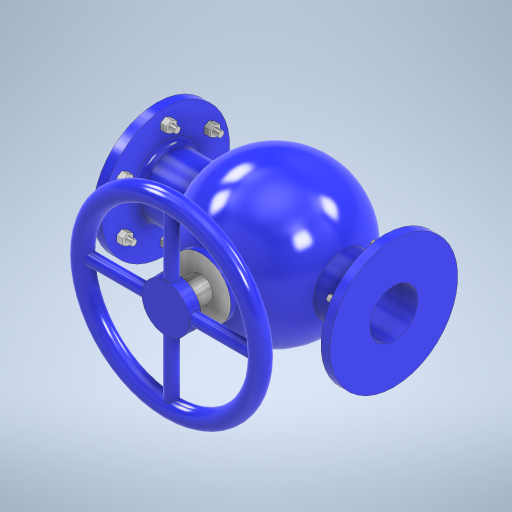
# Autodesk Inventor part: Flansch DN80
Saved by Autodesk Inventor 2023 (Build 270158000, 158)
## iProperties
Created: 2024-11-14
Part Number: Flansch DN80
Material: Generisch
Document SubType Name: Modeling
Designer: aurich
Density: 1 g/cm^3
Appearance: Vorgabe
Author: aurich
Autodesk Inventor part; units mm, degrees
ref_plane "YZ Plane" through (0, 0, 0) normal (1, 0, 0) x (0, 1, 0)
ref_plane "XZ Plane" through (0, 0, 0) normal (0, 1, 0) x (-1, 0, 0)
sketch "Skizze1" plane through (0, 0, 0) normal (1, 0, 0) x (0, 1, 0)
  circle A0 centre (0, 0) radius 40
  circle A1 centre (0, 0) radius 108
  dimension "d0" = 216
  dimension "d1" = 80
  constraints: 2 centre point, 2 coincident
  measures "d0" diameter of A1
  measures "d1" diameter of A0
extrude "Extrusion1" add sketch "Skizze1" along normal blind 15
sketch "Skizze2" plane through (15, 0, 0) normal (1, 0, 0) x (0, 0, -1)
  circle A0 centre (0, 0) radius 40
  circle A1 centre (0, 0) radius 50
  dimension "d4" = 100
  constraints: 2 centre point, 2 coincident
  measures "d4" diameter of A1
extrude "Extrusion2" add sketch "Skizze2" along normal blind 185
fillet "Rundung1" radius 10 1 edges at (15, 0, 50)
sketch "Skizze3" plane through (15, 0, 0) normal (1, 0, 0) x (0, 0, -1)
  circle A0 centre (0, -85) radius 10 construction
  line L0 (0, -95) -> (-8.7647, -89.8146)
  line L1 (-8.7647, -80.1854) -> (0, -75)
  line L2 (0, -75) -> (8.7647, -80.1854)
  line L3 (8.7647, -80.1854) -> (8.7647, -89.8146)
  line L4 (0, -95) -> (8.7647, -89.8146)
  line L5 (-8.7647, -80.1854) -> (-8.7647, -89.8146)
  point P0 (0, 0)
  dimension "d8" = 20
  dimension "d9" = 85
  constraints: 12 end point, 6 point on circle, 2 horizontal alignment, 2 parallel, 2 vertical alignment, 1 centre point, 1 vertical
  measures "d8" diameter of A0
  measures "d9" distance of point (0, 0) A0.centre
extrude "Extrusion3" add sketch "Skizze3" along normal blind 10
sketch "Skizze4" plane through (25, 0, 0) normal (1, 0, 0) x (0, 0, -1)
  circle A0 centre (0, -85) radius 5
  point P0 (0, 0)
  dimension "d12" = 10
  constraints: 1 centre point
  measures "d12" diameter of A0
extrude "Extrusion4" add sketch "Skizze4" along normal blind 10
pattern_circular "Runde Anordnung1" count 6 over 360 about axis through (-10, 0, 0) along (1, 0, 0) of "Extrusion3", "Extrusion4"
mirror "Spiegeln2" about plane through (200, 0, 0) normal (1, 0, 0)
sketch "Skizze5" plane through (0, 0, 0) normal (0, 0, 1) x (1, 0, 0)
  line L0 (0, -108) -> (0, 108) projected
  line L1 (75, 0) -> (325, 0)
  line L2 (375, 50) -> (375, -50) projected
  line L3 (25, 50) -> (25, -50) projected
  arc A0 (15, 60) -> (25, 50) centre (25, 60) ccw projected
  line L4 (25, 50) -> (375, 50) projected
  arc A1 (375, 50) -> (385, 60) centre (375, 60) ccw projected
  line L5 (385, 60) -> (385, 75) projected
  line L6 (385, 108) -> (400, 108) projected
  line L7 (400, 108) -> (400, 40) projected
  line L8 (400, 40) -> (0, 40) projected
  line L9 (0, 40) -> (0, 108) projected
  line L10 (0, 108) -> (15, 108) projected
  line L11 (15, 108) -> (15, 95) projected
  arc A2 (25, -50) -> (15, -60) centre (25, -60) ccw projected
  line L12 (15, -60) -> (15, -75) projected
  line L13 (15, -108) -> (0, -108) projected
  line L14 (0, -108) -> (0, -40) projected
  line L15 (0, -40) -> (400, -40) projected
  line L16 (400, -40) -> (400, -108) projected
  line L17 (400, -108) -> (385, -108) projected
  line L18 (385, -108) -> (385, -95) projected
  arc A3 (385, -60) -> (375, -50) centre (375, -60) ccw projected
  line L19 (375, -50) -> (25, -50) projected
  arc A4 (314.5644, 50) -> (81.5728, 40) centre (200, 0) ccw
  line L20 (-80, 0) -> (480, 0) projected
  line L21 (385, 75) -> (375, 75) projected
  line L22 (375, 75) -> (375, 80) projected
  line L23 (375, 80) -> (365, 80) projected
  line L24 (365, 80) -> (365, 90) projected
  line L25 (365, 90) -> (375, 90) projected
  line L26 (375, 90) -> (375, 95) projected
  line L27 (375, 95) -> (385, 95) projected
  line L28 (385, 95) -> (385, 108) projected
  line L29 (15, 95) -> (25, 95) projected
  line L30 (25, 95) -> (25, 90) projected
  line L31 (25, 90) -> (35, 90) projected
  line L32 (35, 90) -> (35, 80) projected
  line L33 (35, 80) -> (25, 80) projected
  line L34 (25, 80) -> (25, 75) projected
  line L35 (25, 75) -> (15, 75) projected
  line L36 (15, 75) -> (15, 60) projected
  line L37 (15, -75) -> (25, -75) projected
  line L38 (25, -75) -> (25, -80) projected
  line L39 (25, -80) -> (35, -80) projected
  line L40 (35, -80) -> (35, -90) projected
  line L41 (35, -90) -> (25, -90) projected
  line L42 (25, -90) -> (25, -95) projected
  line L43 (25, -95) -> (15, -95) projected
  line L44 (15, -95) -> (15, -108) projected
  line L45 (385, -95) -> (375, -95) projected
  line L46 (375, -95) -> (375, -90) projected
  line L47 (375, -90) -> (365, -90) projected
  line L48 (365, -90) -> (365, -80) projected
  line L49 (365, -80) -> (375, -80) projected
  line L50 (375, -80) -> (375, -75) projected
  line L51 (375, -75) -> (385, -75) projected
  line L52 (385, -75) -> (385, -60) projected
  point P0 (0, 0)
  point P1 (85.4356, 50)
  dimension "d18" = 200
  constraints: 2 end point, 2 point on circle, 2 point on line, 1 centre point, 1 horizontal
  measures "d18" distance from line of L0 A4.centre
revolve "Umdrehung1" add sketch "Skizze5" angle 360 about axis through (-10, 0, 0) along (1, 0, 0) contours A4 L4
ref_plane "Arbeitsebene1" through (200, 0, 125) normal (0, 0, 1) x (1, 0, 0)
sketch "Skizze6" plane through (200, 0, 125) normal (0, 0, 1) x (1, 0, 0)
  circle A0 centre (0, 0) radius 50
  point P0 (-200, 0)
  dimension "d21" = 100
  constraints: 1 centre point
  measures "d21" diameter of A0
extrude "Extrusion5" add sketch "Skizze6" against normal blind 20
sketch "Skizze7" plane through (200, 0, 125) normal (0, 0, 1) x (1, 0, 0)
  circle A0 centre (0, 0) radius 20
  point P0 (-200, 0)
  dimension "d24" = 40
  constraints: 1 centre point
  measures "d24" diameter of A0
extrude "Extrusion6" add sketch "Skizze7" along normal blind 40
sketch "Skizze8" plane through (200, 0, 165) normal (0, 0, 1) x (1, 0, 0)
  arc A0 (28.2843, -28.2843) -> (28.2843, 28.2843) centre (0, 0) ccw
  line L0 (0, 0) -> (28.2843, 28.2843)
  line L1 (0, 0) -> (40, 0) construction
  line L2 (28.2843, 28.2843) -> (0, 0)
  line L3 (28.2843, -28.2843) -> (0, 0)
  line L4 (38.7298, 10) -> (150, 10)
  line L5 (114.5644, -50) -> (114.5644, 50) projected
  line L6 (150, 10) -> (150, -10)
  line L7 (150, -10) -> (38.7298, -10)
  point P0 (-200, 0)
  dimension "d27" = 80
  dimension "d28" = 45
  dimension "d29" = 10
  dimension "d30" = 10
  dimension "d31" = 150
  constraints: 14 end point, 4 point on circle, 3 perpendicular, 1 centre point, 1 collinear, 1 equal length, 1 horizontal, 1 parallel
  measures "d27" diameter of A0
  measures "d28" angle of L1 L0
  measures "d29" distance from line of L0.start L4
  measures "d30" distance from line of L0.start L7
  measures "d31" distance from line of L0.start L6
extrude "Extrusion7" add sketch "Skizze8" along normal blind 20
fillet "Rundung2" radius 10 4 edges at (294.3649, -10, 185) (294.3649, 10, 185) (294.3649, -10, 165) (294.3649, 10, 165)
pattern_circular "Runde Anordnung2" count 4 over 360 about axis through (200, 0, 165) along (0, 0, 1) of "Extrusion7", "Rundung2"
sketch "Skizze9" plane through (0, 0, 0) normal (0, 1, 0) x (-1, 0, 0)
  line L0 (-350, 165) -> (-350, 185) projected
  circle A0 centre (-350, 175) radius 15
  circle A1 centre (-200, 175) radius 10 projected
  line L1 (-200, 185) -> (-200, 206.4235)
  point P0 (0, 0)
  dimension "d38" = 30
  constraints: 2 end point, 1 centre point, 1 midpoint, 1 vertical, 1 vertical alignment, 1 other
  measures "d38" diameter of A0
revolve "Umdrehung2" add sketch "Skizze9" angle 360 about axis through (200, 0, 185) along (0, 0, 1) contours A0
equation "\"d30\" = d29"
